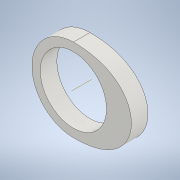
# Autodesk Inventor part: 凸轮（设计）
Saved by Autodesk Inventor 2022 (Build 260153000, 153)
## iProperties
CustomPartVersion: 1
Created: 2023-03-10
Part Number: 凸轮（设计）
Material: Stainless Steel, Austenitic
Document SubType Name: Modeling
Designer: 李承轩
Manufacturer: Standard
Standards Organization: Custom
Density: 1 g/cm^3
Appearance: Steel
Author: 李承轩
Autodesk Inventor part; units mm, degrees
ref_plane "YZ Plane" through (0, 0, 0) normal (1, 0, 0) x (0, 1, 0)
ref_plane "XZ Plane" through (0, 0, 0) normal (0, 1, 0) x (-1, 0, 0)
ref_plane "XY Plane" through (0, 0, 0) normal (0, 0, 1) x (1, 0, 0)
sketch "主草图" plane through (0, 0, 0) normal (0, 0, 1) x (1, 0, 0)
  spline S0 degree 5 poles (0, 25) (0.7436, 25.0058) (2.0459, 24.9856) (4.1649, 24.8981) (6.6383, 24.7115) (9.9572, 24.2779) (12.9872, 23.6878) (16.1276, 22.8402) (19.1517, 21.739) (22.0575, 20.3585) (24.7903, 18.6846) (27.3078, 16.7127) (29.5556, 14.4513) (31.4823, 11.9224) (33.0384, 9.1614) (34.1824, 6.2154) (34.8821, 3.1407) (35.1176, 0) (34.8821, -3.1407) (34.1824, -6.2154) (33.0384, -9.1614) (31.4823, -11.9224) (29.5556, -14.4513) (27.3078, -16.7127) (24.7903, -18.6846) (22.0574, -20.3585) (19.1519, -21.7389) (16.1269, -22.8403) (12.9887, -23.6876) (9.8403, -24.3004) (6.5695, -24.7185) (3.5422, -24.943) (0.0519, -25.052) (-2.4149, -24.9589) (-5.1951, -24.5298) (-7.721, -23.8479) (-10.2022, -22.9006) (-12.5318, -21.7104) (-14.7361, -20.2808) (-16.7737, -18.6297) (-18.6298, -16.7742) (-20.2809, -14.735) (-21.7101, -12.5343) (-22.9013, -10.1963) (-23.8417, -7.7466) (-24.5208, -5.2121) (-24.9313, -2.6204) (-25.0686, 0) (-24.9313, 2.6204) (-24.5208, 5.2121) (-23.8417, 7.7466) (-22.9013, 10.1963) (-21.7101, 12.5343) (-20.2808, 14.735) (-18.6299, 16.7742) (-16.7735, 18.6297) (-14.7365, 20.2808) (-12.5308, 21.7105) (-10.2044, 22.9004) (-7.827, 23.8061) (-5.3545, 24.4918) (-3.1793, 24.8426) (-1.7184, 24.9625) (-0.6635, 24.9948) (0, 25) knots 0 0 0 0 0 0 0.021287 0.03545 0.05313 0.070768 0.088362 0.105917 0.123437 0.140928 0.15839 0.175824 0.193228 0.210602 0.227951 0.245279 0.262597 0.279914 0.297243 0.314591 0.331966 0.34937 0.366804 0.384266 0.401756 0.419277 0.436831 0.454425 0.472063 0.489743 0.507072 0.524039 0.540634 0.556847 0.572674 0.588501 0.604328 0.620155 0.635982 0.651809 0.667635 0.683462 0.699289 0.715116 0.730943 0.74677 0.762597 0.778424 0.794251 0.810077 0.825904 0.841731 0.857558 0.873385 0.889212 0.905039 0.920866 0.936692 0.952519 0.968346 0.981008 1 1 1 1 1 1
  point P0 (6.5702, 24.6757)
  point P1 (9.8108, 24.2515)
  point P2 (12.9988, 23.6256)
  point P3 (16.1148, 22.7719)
  point P4 (19.1343, 21.664)
  point P5 (22.0248, 20.2795)
  point P6 (24.7457, 18.6037)
  point P7 (27.2491, 16.6327)
  point P8 (29.4834, 14.3753)
  point P9 (31.3964, 11.8542)
  point P10 (32.9402, 9.1052)
  point P11 (34.0739, 6.1752)
  point P12 (34.7669, 3.1197)
  point P13 (35, 0)
  point P14 (34.7669, -3.1197)
  point P15 (34.0739, -6.1752)
  point P16 (32.9402, -9.1052)
  point P17 (31.3964, -11.8542)
  point P18 (29.4834, -14.3753)
  point P19 (27.2491, -16.6327)
  point P20 (24.7457, -18.6037)
  point P21 (22.0248, -20.2795)
  point P22 (19.1343, -21.664)
  point P23 (16.1148, -22.7719)
  point P24 (12.9988, -23.6256)
  point P25 (9.8108, -24.2515)
  point P26 (6.5702, -24.6757)
  point P27 (3.2942, -24.9202)
  point P28 (0, -25)
  point P29 (-2.6132, -24.863)
  point P30 (-5.1978, -24.4537)
  point P31 (-7.7254, -23.7764)
  point P32 (-10.1684, -22.8386)
  point P33 (-12.5, -21.6506)
  point P34 (-14.6946, -20.2254)
  point P35 (-16.7283, -18.5786)
  point P36 (-18.5786, -16.7283)
  point P37 (-20.2254, -14.6946)
  point P38 (-21.6506, -12.5)
  point P39 (-22.8386, -10.1684)
  point P40 (-23.7764, -7.7254)
  point P41 (-24.4537, -5.1978)
  point P42 (-24.863, -2.6132)
  point P43 (-25, 0)
  point P44 (-24.863, 2.6132)
  point P45 (-24.4537, 5.1978)
  point P46 (-23.7764, 7.7254)
  point P47 (-22.8386, 10.1684)
  point P48 (-21.6506, 12.5)
  point P49 (-20.2254, 14.6946)
  point P50 (-18.5786, 16.7283)
  point P51 (-16.7283, 18.5786)
  point P52 (-14.6946, 20.2254)
  point P53 (-12.5, 21.6506)
  point P54 (-10.1684, 22.8386)
  point P55 (-7.7254, 23.7764)
  point P56 (-5.1978, 24.4537)
  point P57 (-2.6132, 24.863)
  constraints: 60 other
extrude "凸轮" add sketch "主草图" along normal blind 10
sketch "草图2" plane through (0, 0, 10) normal (0, 0, 1) x (1, 0, 0)
  circle A0 centre (0, 0) radius 20
  dimension "d4" = 40
  constraints: 1 centre point, 1 coincident
  measures "d4" diameter of A0
extrude "拉伸2" cut sketch "草图2" against normal through all
body "Solid1"
